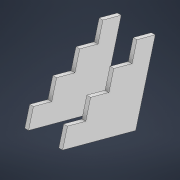
# Autodesk Inventor part: 階梯2
Saved by Autodesk Inventor 2021 (Build 250183000, 183)
## iProperties
Created: 2020-12-28
Part Number: 階梯2
Material: 一般
Document SubType Name: Modeling
Designer: zihon
Density: 1 g/cm^3
Appearance: 預設
Author: zihon
Autodesk Inventor part; units mm, degrees
ref_plane "YZ Plane" through (0, 0, 0) normal (1, 0, 0) x (0, 1, 0)
ref_plane "XZ Plane" through (0, 0, 0) normal (0, 1, 0) x (-1, 0, 0)
ref_plane "XY Plane" through (0, 0, 0) normal (0, 0, 1) x (1, 0, 0)
sketch "草圖1" plane through (0, 0, 0) normal (1, 0, 0) x (0, 1, 0)
  line L0 (0.483, -1.0953) -> (0.3536, -1.5783)
  line L1 (-0.6711, 0) -> (2.2147, 0) projected
  line L2 (0.7418, -0.1294) -> (0.6124, -0.6124)
  line L3 (0.6124, -0.6124) -> (1.0953, -0.7418)
  line L4 (1.0953, -0.7418) -> (0.9659, -1.2247)
  line L5 (0.9659, -1.2247) -> (1.4489, -1.3542)
  line L6 (0, -2.9394) -> (0, 0.4899) projected
  line L7 (1.4489, -1.3542) -> (1.3195, -1.8371)
  line L8 (1.3195, -1.8371) -> (1.8024, -1.9665)
  line L9 (1.8024, -1.9665) -> (1.673, -2.4495)
  line L10 (0.483, -1.0953) -> (0, -0.9659)
  line L11 (0.7418, -0.1294) -> (0.2588, 0)
  line L12 (0.2588, 0) -> (0, -0.9659)
  line L13 (0, -0.9659) -> (0.1294, -0.483)
  line L14 (0.1294, -0.483) -> (0.1294, -0.483)
  line L15 (0.3536, -1.5783) -> (0.8365, -1.7077)
  line L16 (0.8365, -1.7077) -> (0.7071, -2.1907)
  line L17 (0.7071, -2.1907) -> (1.673, -2.4495)
  line L18 (0.7071, -2.1907) -> (-0.2588, -1.9319)
  line L19 (-0.2588, -1.9319) -> (0, -0.9659)
  point P0 (0, 0)
  dimension "d28" = 0.5
  dimension "d29" = 0.5
  dimension "d34" = 0.5
  dimension "d43" = 0.5
  dimension "d48" = 0.5
  dimension "d49" = 15
  dimension "d50" = 0.5
  dimension "d52" = 0.5
  dimension "d53" = 0.5
  constraints: 36 end point, 15 perpendicular, 5 parallel, 3 point on line, 1 collinear, 1 midpoint
  measures "d28" distance of L2.start L2.end
  measures "d29" distance between parallel lines of L0 L4
  measures "d34" distance of L2.end L3.end
  measures "d43" distance of L0.start L0.end
  measures "d48" distance of L2.start L11.end
  measures "d49" angle of L1 L11
  measures "d50" distance between parallel lines of L13 L2
  measures "d52" distance of L0.end L15.end
  measures "d53" distance of L15.end L16.end
extrude "擠出1" add sketch "草圖1" along normal mid plane 1 contours L10 L12 L11 L2 L3 L4 L5 L7 L8 L9 L17 L16 L15 L0 | L0 L15 L16 L18 L6 L10 | L6 L18 L19
sketch "草圖3" plane through (0, 0, 0) normal (0, 0, 1) x (1, 0, 0)
  line L0 (-0.4, 1.8024) -> (0.4, 1.8024)
  line L1 (0.4, 1.8024) -> (0.4, -0.2588)
  line L2 (0.4, -0.2588) -> (-0.4, -0.2588)
  line L3 (-0.4, -0.2588) -> (-0.4, 1.8024)
  line L4 (-0.4, 1.8024) -> (0.4, -0.2588) construction
  line L5 (0.4, 1.8024) -> (-0.4, -0.2588) construction
  line L6 (0, -0.3605) -> (0, 2.1629) projected
  line L7 (-0.7, 0) -> (0.7, 0) projected
  line L8 (-0.5, 1.8024) -> (0.5, 1.8024) projected
  line L9 (-0.5, -0.2588) -> (0.5, -0.2588) projected
  point P0 (0, 0)
  point P1 (0, 0.7718)
  point P2 (0, 0.7718)
  point P3 (-0.7, 0)
  point P4 (0.7, 0)
  dimension "d21" = 0.8
  constraints: 12 end point, 3 midpoint, 2 collinear, 2 parallel, 1 horizontal, 1 perpendicular, 1 point on line, 1 other
  measures "d21" distance between parallel lines of L1 L3
extrude "擠出3" cut sketch "草圖3" against normal blind 10
